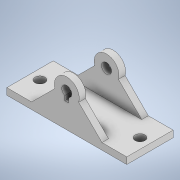
# Autodesk Inventor part: Top_Pulley
Saved by Autodesk Inventor 2020 (Build 240168000, 168)
## iProperties
Created: 2019-09-27
Part Number: Top_Pulley
Material: 일반
Document SubType Name: Modeling
Designer: Knowblesse
Density: 1 g/cm^3
Appearance: 기본값
Author: Knowblesse
## iProperties of the stored document _3D 인쇄.ipt
Created: 2019-09-27
Part Number: _3D 인쇄
Material: 일반
Document SubType Name: Modeling
Designer: Knowblesse
Density: 1 g/cm^3
Appearance: 기본값
Author: Knowblesse
Autodesk Inventor part; units mm, degrees
ref_plane "YZ Plane" through (0, 0, 0) normal (1, 0, 0) x (0, 1, 0)
ref_plane "XZ Plane" through (0, 0, 0) normal (0, 1, 0) x (-1, 0, 0)
ref_plane "XY Plane" through (0, 0, 0) normal (0, 0, 1) x (1, 0, 0)
sketch "스케치1" plane through (0, 0, 0) normal (0, 0, 1) x (1, 0, 0)
  line L0 (0, 0) -> (21.2132, 21.2132)
  line L1 (0, 0) -> (30, 0) construction
  line L2 (21.2132, 21.2132) -> (42.4264, 0)
  line L3 (42.4264, 0) -> (0, 0)
  circle A0 centre (21.2132, 16.2132) radius 7.5
  circle A1 centre (21.2132, 16.2132) radius 3.05
  point P0 (14.0361, 14.0361)
  point P1 (28.3903, 14.0361)
  dimension "d0" = 30
  dimension "d1" = 45
  dimension "d2" = 30
  dimension "d3" = 90
  dimension "d4" = 15
  dimension "d5" = 5
  dimension "d6" = 6.1
  constraints: 8 end point, 2 centre point, 1 coincident, 1 equal length, 1 horizontal, 1 perpendicular, 1 vertical alignment
  measures "d0" distance of L0.start L0.end
  measures "d1" angle of L1 L0
  measures "d2" distance of L0.end L2.end
  measures "d3" angle of L0 L2
  measures "d4" diameter of A0
  measures "d5" distance of L0.end A0.centre
  measures "d6" diameter of A1
extrude "돌출1" add sketch "스케치1" along normal blind 4
sketch "스케치2" plane through (0, 0, 0) normal (0, -1, 0) x (1, 0, 0)
  line L0 (57.4264, 14) -> (-15, 14)
  line L1 (-15, 14) -> (-15, 0)
  line L2 (-15, 0) -> (57.4264, 0)
  line L3 (57.4264, 0) -> (57.4264, 14)
  line L4 (42.4264, 0) -> (42.4264, 4) projected
  line L5 (0, 0) -> (0, 4) projected
  line L6 (0, 0) -> (42.4264, 0) projected
  dimension "d9" = 14
  dimension "d10" = 15
  dimension "d11" = 15
  constraints: 8 end point, 2 parallel, 1 collinear, 1 horizontal, 1 perpendicular
  measures "d9" distance between parallel lines of L0 L6
  measures "d10" distance between parallel lines of L4 L3
  measures "d11" distance between parallel lines of L5 L1
extrude "돌출2" add sketch "스케치2" along normal blind 4
mirror "미러1" about plane through (57.4264, 0, 14) normal (0, 0, 1) of "돌출1", "돌출2"
sketch "스케치3" plane through (0, 0, 0) normal (0, 1, 0) x (1, 0, 0)
  line L0 (57.4264, 0) -> (57.4264, -28) projected
  line L1 (-15, 0) -> (-15, -28) projected
  point P0 (0, 0)
  point P1 (51.4264, -14)
  point P2 (-9, -14)
  point P3 (57.4264, -14)
  dimension "d14" = 6
  dimension "d15" = 6
  constraints: 2 horizontal alignment, 1 midpoint
  measures "d14" distance from line of L0 point (51.426, -14)
  measures "d15" distance from line of L1 point (-9, -14)
hole "구멍1" at (51.4264, 0, 14) at (-9, 0, 14) direction (0, -1, 0) diameter 6 end through all
sketch "스케치4" plane through (21.2132, 16.2132, 28) normal (0, 0, 1) x (1, 0, 0)
  circle A0 centre (0, 0) radius 3.05 projected
  line L0 (-1.2, -2.55) -> (1.2, -2.55)
  line L1 (1.2, -2.55) -> (1.2, -5.55)
  line L2 (1.2, -5.55) -> (-1.2, -5.55)
  line L3 (-1.2, -5.55) -> (-1.2, -2.55)
  point P0 (-21.2132, -16.2132)
  point P1 (0, -3.05)
  dimension "d23" = 2.4
  dimension "d24" = 3
  dimension "d27" = 0.5
  constraints: 8 end point, 2 parallel, 2 vertical alignment, 1 horizontal, 1 perpendicular, 1 other
  measures "d23" distance of L1.end L2.end
  measures "d24" distance of L0.end L1.end
  measures "d27" distance from line of L0 point (0, -3.05)
extrude "돌출3" cut sketch "스케치4" against normal blind 4 contours L3 L0 L1 A0 | A0 L1 L2 L3 picked at (0, -2.7167)
